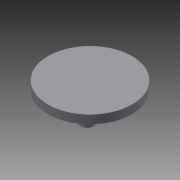
# Autodesk Inventor part: PSteg
Saved by Autodesk Inventor 2014 (Build 180170000, 170)
## iProperties
Created: 2013-05-23
Part Number: PSteg
Material: Generisch
Document SubType Name: Modeling
Designer: hartmann
Density: 1 g/cm^3
Appearance: Vorgabe
Author: hartmann
Autodesk Inventor part; units mm, degrees
ref_plane "YZ Plane" through (0, 0, 0) normal (1, 0, 0) x (0, 1, 0)
ref_plane "XZ Plane" through (0, 0, 0) normal (0, 1, 0) x (-1, 0, 0)
ref_plane "XY Plane" through (0, 0, 0) normal (0, 0, 1) x (1, 0, 0)
sketch "Skizze1" plane through (0, 0, 0) normal (0, 0, 1) x (1, 0, 0)
  arc A0 (1.0212, 1.5725) -> (1.1577, 2.2721) centre (-0.9647, 2.323) ccw projected
  arc A1 (1.1577, 2.2721) -> (0.9138, 2.3806) centre (0, 0) ccw projected
  arc A2 (0.9138, 2.3806) -> (0.4853, 1.8111) centre (2.3719, 0.8375) ccw projected
  arc A3 (0.4853, 1.8111) -> (0.2933, 1.8519) centre (0, 0) ccw projected
  arc A4 (0.2933, 1.8519) -> (0.1335, 2.5465) centre (-1.8262, 1.7298) ccw projected
  arc A5 (0.1335, 2.5465) -> (-0.1335, 2.5465) centre (0, 0) ccw projected
  arc A6 (-0.1335, 2.5465) -> (-0.2933, 1.8519) centre (1.8262, 1.7298) ccw projected
  arc A7 (-0.2933, 1.8519) -> (-0.4853, 1.8111) centre (0, 0) ccw projected
  arc A8 (-0.4853, 1.8111) -> (-0.9138, 2.3806) centre (-2.3719, 0.8375) ccw projected
  arc A9 (-0.9138, 2.3806) -> (-1.1577, 2.2721) centre (0, 0) ccw projected
  arc A10 (-1.1577, 2.2721) -> (-1.0212, 1.5725) centre (0.9647, 2.323) ccw projected
  arc A11 (-1.0212, 1.5725) -> (-1.18, 1.4571) centre (0, 0) ccw projected
  arc A12 (-1.18, 1.4571) -> (-1.8031, 1.8031) centre (-2.5074, -0.1996) ccw projected
  arc A13 (-1.8031, 1.8031) -> (-1.9817, 1.6048) centre (0, 0) ccw projected
  arc A14 (-1.9817, 1.6048) -> (-1.5725, 1.0212) centre (-0.0636, 2.5146) ccw projected
  arc A15 (-1.5725, 1.0212) -> (-1.6706, 0.8512) centre (0, 0) ccw projected
  arc A16 (-1.6706, 0.8512) -> (-2.3806, 0.9138) centre (-2.2095, -1.2022) ccw projected
  arc A17 (-2.3806, 0.9138) -> (-2.4631, 0.66) centre (0, 0) ccw projected
  arc A18 (-2.4631, 0.66) -> (-1.8519, 0.2933) centre (-1.0808, 2.2713) ccw projected
  arc A19 (-1.8519, 0.2933) -> (-1.8724, 0.0981) centre (0, 0) ccw projected
  arc A20 (-1.8724, 0.0981) -> (-2.5465, -0.1335) centre (-1.5295, -1.997) ccw projected
  arc A21 (-2.5465, -0.1335) -> (-2.5186, -0.3989) centre (0, 0) ccw projected
  arc A22 (-2.5186, -0.3989) -> (-1.8111, -0.4853) centre (-1.9112, 1.6353) ccw projected
  arc A23 (-1.8111, -0.4853) -> (-1.7505, -0.6719) centre (0, 0) ccw projected
  arc A24 (-1.7505, -0.6719) -> (-2.2721, -1.1577) centre (-0.585, -2.4464) ccw projected
  arc A25 (-2.2721, -1.1577) -> (-2.1386, -1.3888) centre (0, 0) ccw projected
  arc A26 (-2.1386, -1.3888) -> (-1.4571, -1.18) centre (-2.4111, 0.7166) ccw projected
  arc A27 (-1.4571, -1.18) -> (-1.3258, -1.3258) centre (0, 0) ccw projected
  arc A28 (-1.3258, -1.3258) -> (-1.6048, -1.9817) centre (0.4606, -2.4728) ccw projected
  arc A29 (-1.6048, -1.9817) -> (-1.3888, -2.1386) centre (0, 0) ccw projected
  arc A30 (-1.3888, -2.1386) -> (-0.8512, -1.6706) centre (-2.4942, -0.3261) ccw projected
  arc A31 (-0.8512, -1.6706) -> (-0.6719, -1.7505) centre (0, 0) ccw projected
  arc A32 (-0.6719, -1.7505) -> (-0.66, -2.4631) centre (1.4266, -2.0717) ccw projected
  arc A33 (-0.66, -2.4631) -> (-0.3989, -2.5186) centre (0, 0) ccw projected
  arc A34 (-0.3989, -2.5186) -> (-0.0981, -1.8724) centre (-2.1459, -1.3123) ccw projected
  arc A35 (-0.0981, -1.8724) -> (0.0981, -1.8724) centre (0, 0) ccw projected
  arc A36 (0.0981, -1.8724) -> (0.3989, -2.5186) centre (2.1459, -1.3123) ccw projected
  arc A37 (0.3989, -2.5186) -> (0.66, -2.4631) centre (0, 0) ccw projected
  arc A38 (0.66, -2.4631) -> (0.6719, -1.7505) centre (-1.4266, -2.0717) ccw projected
  arc A39 (0.6719, -1.7505) -> (0.8512, -1.6706) centre (0, 0) ccw projected
  arc A40 (0.8512, -1.6706) -> (1.3888, -2.1386) centre (2.4942, -0.3261) ccw projected
  arc A41 (1.3888, -2.1386) -> (1.6048, -1.9817) centre (0, 0) ccw projected
  arc A42 (1.6048, -1.9817) -> (1.3258, -1.3258) centre (-0.4606, -2.4728) ccw projected
  arc A43 (1.3258, -1.3258) -> (1.4571, -1.18) centre (0, 0) ccw projected
  arc A44 (1.4571, -1.18) -> (2.1386, -1.3888) centre (2.4111, 0.7166) ccw projected
  arc A45 (2.1386, -1.3888) -> (2.2721, -1.1577) centre (0, 0) ccw projected
  arc A46 (2.2721, -1.1577) -> (1.7505, -0.6719) centre (0.585, -2.4464) ccw projected
  arc A47 (1.7505, -0.6719) -> (1.8111, -0.4853) centre (0, 0) ccw projected
  arc A48 (1.8111, -0.4853) -> (2.5186, -0.3989) centre (1.9112, 1.6353) ccw projected
  arc A49 (2.5186, -0.3989) -> (2.5465, -0.1335) centre (0, 0) ccw projected
  arc A50 (2.5465, -0.1335) -> (1.8724, 0.0981) centre (1.5295, -1.997) ccw projected
  arc A51 (1.8724, 0.0981) -> (1.8519, 0.2933) centre (0, 0) ccw projected
  arc A52 (1.8519, 0.2933) -> (2.4631, 0.66) centre (1.0808, 2.2713) ccw projected
  arc A53 (2.4631, 0.66) -> (2.3806, 0.9138) centre (0, 0) ccw projected
  arc A54 (2.3806, 0.9138) -> (1.6706, 0.8512) centre (2.2095, -1.2022) ccw projected
  arc A55 (1.6706, 0.8512) -> (1.5725, 1.0212) centre (0, 0) ccw projected
  arc A56 (1.5725, 1.0212) -> (1.9817, 1.6048) centre (0.0636, 2.5146) ccw projected
  arc A57 (1.9817, 1.6048) -> (1.8031, 1.8031) centre (0, 0) ccw projected
  arc A58 (1.8031, 1.8031) -> (1.18, 1.4571) centre (2.5074, -0.1996) ccw projected
  arc A59 (1.18, 1.4571) -> (1.0212, 1.5725) centre (0, 0) ccw projected
  circle A60 centre (0, 0) radius 10
  dimension "d0" = 20
  constraints: 1 centre point, 1 coincident
  measures "d0" diameter of A60
extrude "Extrusion1" add sketch "Skizze1" along normal blind 2 contours A59 A58 A57 A56 A55 A54 A53 A52 A51 A50 A49 A48 A47 A46 A45 A44 A43 A42 A41 A40 A39 A38 A37 A36 A35 A34 A33 A32 A31 A30 A29 A28 A27 A26 A25 A24 A23 A22 A21 A20 A19 A18 A17 A16 A15 A14 A13 A12 A11 A10 A9 A8 A7 A6 A5 A4 A3 A2 A1 A0 | A60
sketch "Skizze2" plane through (0, 0, 0) normal (0, 0, -1) x (-1, 0, 0)
  circle A0 centre (-2.2201, 6.3744) radius 1.5 projected
  arc A1 (-5.5549, 8.8024) -> (-6.2431, 8.9928) centre (-6.6934, 6.0252) ccw projected
  arc A2 (-6.2431, 8.9928) -> (-6.3746, 8.7787) centre (-2.2201, 6.3744) ccw projected
  arc A3 (-6.3746, 8.7787) -> (-5.8936, 8.2509) centre (-3.9314, 10.5222) ccw projected
  arc A4 (-5.8936, 8.2509) -> (-5.9868, 8.056) centre (-2.2201, 6.3744) ccw projected
  arc A5 (-5.9868, 8.056) -> (-6.6996, 8.0992) centre (-6.5231, 5.1028) ccw projected
  arc A6 (-6.6996, 8.0992) -> (-6.7837, 7.8624) centre (-2.2201, 6.3744) ccw projected
  arc A7 (-6.7837, 7.8624) -> (-6.2035, 7.4461) centre (-4.7564, 10.0758) ccw projected
  arc A8 (-6.2035, 7.4461) -> (-6.2541, 7.2362) centre (-2.2201, 6.3744) ccw projected
  arc A9 (-6.2541, 7.2362) -> (-6.9603, 7.1301) centre (-6.1647, 4.236) ccw projected
  arc A10 (-6.9603, 7.1301) -> (-6.9933, 6.881) centre (-2.2201, 6.3744) ccw projected
  arc A11 (-6.9933, 6.881) -> (-6.3393, 6.5945) centre (-5.4705, 9.4676) ccw projected
  arc A12 (-6.3393, 6.5945) -> (-6.3451, 6.3786) centre (-2.2201, 6.3744) ccw projected
  arc A13 (-6.3451, 6.3786) -> (-7.0138, 6.1281) centre (-5.6339, 3.4626) ccw projected
  arc A14 (-7.0138, 6.1281) -> (-6.9944, 5.8775) centre (-2.2201, 6.3744) ccw projected
  arc A15 (-6.9944, 5.8775) -> (-6.295, 5.7333) centre (-6.0426, 8.7242) ccw projected
  arc A16 (-6.295, 5.7333) -> (-6.2559, 5.5209) centre (-2.2201, 6.3744) ccw projected
  arc A17 (-6.2559, 5.5209) -> (-6.8578, 5.1368) centre (-4.9539, 2.8165) ccw projected
  arc A18 (-6.8578, 5.1368) -> (-6.7867, 4.8958) centre (-2.2201, 6.3744) ccw projected
  arc A19 (-6.7867, 4.8958) -> (-6.0727, 4.9001) centre (-6.4476, 7.8781) ccw projected
  arc A20 (-6.0727, 4.9001) -> (-5.9902, 4.7005) centre (-2.2201, 6.3744) ccw projected
  arc A21 (-5.9902, 4.7005) -> (-6.4992, 4.1996) centre (-4.1544, 2.3259) ccw projected
  arc A22 (-6.4992, 4.1996) -> (-6.3795, 3.9787) centre (-2.2201, 6.3744) ccw projected
  arc A23 (-6.3795, 3.9787) -> (-5.6819, 4.1313) centre (-6.6678, 6.9663) ccw projected
  arc A24 (-5.6819, 4.1313) -> (-5.5598, 3.9532) centre (-2.2201, 6.3744) ccw projected
  arc A25 (-5.5598, 3.9532) -> (-5.9535, 3.3575) centre (-3.2704, 2.0122) ccw projected
  arc A26 (-5.9535, 3.3575) -> (-5.7905, 3.1662) centre (-2.2201, 6.3744) ccw projected
  arc A27 (-5.7905, 3.1662) -> (-5.1399, 3.4606) centre (-6.6937, 6.0286) ccw projected
  arc A28 (-5.1399, 3.4606) -> (-4.9834, 3.3118) centre (-2.2201, 6.3744) ccw projected
  arc A29 (-4.9834, 3.3118) -> (-5.2447, 2.6472) centre (-2.3404, 1.8891) ccw projected
  arc A30 (-5.2447, 2.6472) -> (-5.0455, 2.494) centre (-2.2201, 6.3744) ccw projected
  arc A31 (-5.0455, 2.494) -> (-4.4703, 2.9172) centre (-6.524, 5.1061) ccw projected
  arc A32 (-4.4703, 2.9172) -> (-4.2863, 2.8042) centre (-2.2201, 6.3744) ccw projected
  arc A33 (-4.2863, 2.8042) -> (-4.4036, 2.0998) centre (-1.4053, 1.9622) ccw projected
  arc A34 (-4.4036, 2.0998) -> (-4.1769, 1.9914) centre (-2.2201, 6.3744) ccw projected
  arc A35 (-4.1769, 1.9914) -> (-3.7023, 2.5249) centre (-6.1663, 4.239) ccw projected
  arc A36 (-3.7023, 2.5249) -> (-3.4988, 2.4526) centre (-2.2201, 6.3744) ccw projected
  arc A37 (-3.4988, 2.4526) -> (-3.4672, 1.7393) centre (-0.5057, 2.228) ccw projected
  arc A38 (-3.4672, 1.7393) -> (-3.2229, 1.6803) centre (-2.2201, 6.3744) ccw projected
  arc A39 (-3.2229, 1.6803) -> (-2.8696, 2.3009) centre (-5.6361, 3.4652) ccw projected
  arc A40 (-2.8696, 2.3009) -> (-2.6555, 2.2725) centre (-2.2201, 6.3744) ccw projected
  arc A41 (-2.6555, 2.2725) -> (-2.4762, 1.5813) centre (0.3189, 2.6751) ccw projected
  arc A42 (-2.4762, 1.5813) -> (-2.225, 1.5744) centre (-2.2201, 6.3744) ccw projected
  arc A43 (-2.225, 1.5744) -> (-2.0084, 2.2549) centre (-4.9566, 2.8186) ccw projected
  arc A44 (-2.0084, 2.2549) -> (-1.7931, 2.2716) centre (-2.2201, 6.3744) ccw projected
  arc A45 (-1.7931, 2.2716) -> (-1.4741, 1.6328) centre (1.0326, 3.2838) ccw projected
  arc A46 (-1.4741, 1.6328) -> (-1.2269, 1.6783) centre (-2.2201, 6.3744) ccw projected
  arc A47 (-1.2269, 1.6783) -> (-1.1566, 2.3889) centre (-4.1575, 2.3273) ccw projected
  arc A48 (-1.1566, 2.3889) -> (-0.9494, 2.45) centre (-2.2201, 6.3744) ccw projected
  arc A49 (-0.9494, 2.45) -> (-0.5045, 1.8915) centre (1.6041, 4.0276) ccw projected
  arc A50 (-0.5045, 1.8915) -> (-0.2723, 1.9874) centre (-2.2201, 6.3744) ccw projected
  arc A51 (-0.2723, 1.9874) -> (-0.3512, 2.6971) centre (-3.2737, 2.013) ccw projected
  arc A52 (-0.3512, 2.6971) -> (-0.1613, 2.8) centre (-2.2201, 6.3744) ccw projected
  arc A53 (-0.1613, 2.8) -> (0.39, 2.3462) centre (2.0084, 4.874) ccw projected
  arc A54 (0.39, 2.3462) -> (0.5973, 2.4883) centre (-2.2201, 6.3744) ccw projected
  arc A55 (0.5973, 2.4883) -> (0.3725, 3.1661) centre (-2.3439, 1.8892) ccw projected
  arc A56 (0.3725, 3.1661) -> (0.5369, 3.3062) centre (-2.2201, 6.3744) ccw projected
  arc A57 (0.5369, 3.3062) -> (1.1705, 2.9769) centre (2.228, 5.786) ccw projected
  arc A58 (1.1705, 2.9769) -> (1.3437, 3.159) centre (-2.2201, 6.3744) ccw projected
  arc A59 (1.3437, 3.159) -> (0.9829, 3.7752) centre (-1.4086, 1.9615) ccw projected
  arc A60 (0.9829, 3.7752) -> (1.1146, 3.9464) centre (-2.2201, 6.3744) ccw projected
  arc A61 (1.1146, 3.9464) -> (1.8028, 3.7561) centre (2.2531, 6.7236) ccw projected
  arc A62 (1.8028, 3.7561) -> (1.9343, 3.9702) centre (-2.2201, 6.3744) ccw projected
  arc A63 (1.9343, 3.9702) -> (1.4534, 4.498) centre (-0.5089, 2.2267) ccw projected
  arc A64 (1.4534, 4.498) -> (1.5465, 4.6928) centre (-2.2201, 6.3744) ccw projected
  arc A65 (1.5465, 4.6928) -> (2.2593, 4.6497) centre (2.0828, 7.6461) ccw projected
  arc A66 (2.2593, 4.6497) -> (2.3434, 4.8865) centre (-2.2201, 6.3744) ccw projected
  arc A67 (2.3434, 4.8865) -> (1.7632, 5.3028) centre (0.3161, 2.6731) ccw projected
  arc A68 (1.7632, 5.3028) -> (1.8138, 5.5127) centre (-2.2201, 6.3744) ccw projected
  arc A69 (1.8138, 5.5127) -> (2.52, 5.6187) centre (1.7244, 8.5129) ccw projected
  arc A70 (2.52, 5.6187) -> (2.553, 5.8679) centre (-2.2201, 6.3744) ccw projected
  arc A71 (2.553, 5.8679) -> (1.899, 6.1544) centre (1.0302, 3.2813) ccw projected
  arc A72 (1.899, 6.1544) -> (1.9049, 6.3703) centre (-2.2201, 6.3744) ccw projected
  arc A73 (1.9049, 6.3703) -> (2.5735, 6.6208) centre (1.1936, 9.2863) ccw projected
  arc A74 (2.5735, 6.6208) -> (2.5541, 6.8713) centre (-2.2201, 6.3744) ccw projected
  arc A75 (2.5541, 6.8713) -> (1.8547, 7.0156) centre (1.6023, 4.0247) ccw projected
  arc A76 (1.8547, 7.0156) -> (1.8156, 7.228) centre (-2.2201, 6.3744) ccw projected
  arc A77 (1.8156, 7.228) -> (2.4176, 7.6121) centre (0.5136, 9.9324) ccw projected
  arc A78 (2.4176, 7.6121) -> (2.3464, 7.8531) centre (-2.2201, 6.3744) ccw projected
  arc A79 (2.3464, 7.8531) -> (1.6324, 7.8488) centre (2.0073, 4.8708) ccw projected
  arc A80 (1.6324, 7.8488) -> (1.5499, 8.0484) centre (-2.2201, 6.3744) ccw projected
  arc A81 (1.5499, 8.0484) -> (2.0589, 8.5492) centre (-0.2859, 10.423) ccw projected
  arc A82 (2.0589, 8.5492) -> (1.9392, 8.7702) centre (-2.2201, 6.3744) ccw projected
  arc A83 (1.9392, 8.7702) -> (1.2416, 8.6176) centre (2.2275, 5.7826) ccw projected
  arc A84 (1.2416, 8.6176) -> (1.1195, 8.7957) centre (-2.2201, 6.3744) ccw projected
  arc A85 (1.1195, 8.7957) -> (1.5132, 9.3914) centre (-1.1699, 10.7367) ccw projected
  arc A86 (1.5132, 9.3914) -> (1.3502, 9.5826) centre (-2.2201, 6.3744) ccw projected
  arc A87 (1.3502, 9.5826) -> (0.6996, 9.2883) centre (2.2534, 6.7202) ccw projected
  arc A88 (0.6996, 9.2883) -> (0.5431, 9.4371) centre (-2.2201, 6.3744) ccw projected
  arc A89 (0.5431, 9.4371) -> (0.8044, 10.1017) centre (-2.0998, 10.8597) ccw projected
  arc A90 (0.8044, 10.1017) -> (0.6052, 10.2549) centre (-2.2201, 6.3744) ccw projected
  arc A91 (0.6052, 10.2549) -> (0.03, 9.8317) centre (2.0838, 7.6428) ccw projected
  arc A92 (0.03, 9.8317) -> (-0.154, 9.9447) centre (-2.2201, 6.3744) ccw projected
  arc A93 (-0.154, 9.9447) -> (-0.0367, 10.6491) centre (-3.035, 10.7867) ccw projected
  arc A94 (-0.0367, 10.6491) -> (-0.2634, 10.7575) centre (-2.2201, 6.3744) ccw projected
  arc A95 (-0.2634, 10.7575) -> (-0.738, 10.224) centre (1.726, 8.5099) ccw projected
  arc A96 (-0.738, 10.224) -> (-0.9415, 10.2962) centre (-2.2201, 6.3744) ccw projected
  arc A97 (-0.9415, 10.2962) -> (-0.9731, 11.0096) centre (-3.9346, 10.5209) ccw projected
  arc A98 (-0.9731, 11.0096) -> (-1.2174, 11.0685) centre (-2.2201, 6.3744) ccw projected
  arc A99 (-1.2174, 11.0685) -> (-1.5707, 10.448) centre (1.1958, 9.2837) ccw projected
  arc A100 (-1.5707, 10.448) -> (-1.7848, 10.4764) centre (-2.2201, 6.3744) ccw projected
  arc A101 (-1.7848, 10.4764) -> (-1.9641, 11.1676) centre (-4.7592, 10.0738) ccw projected
  arc A102 (-1.9641, 11.1676) -> (-2.2153, 11.1744) centre (-2.2201, 6.3744) ccw projected
  arc A103 (-2.2153, 11.1744) -> (-2.4319, 10.494) centre (0.5163, 9.9303) ccw projected
  arc A104 (-2.4319, 10.494) -> (-2.6472, 10.4773) centre (-2.2201, 6.3744) ccw projected
  arc A105 (-2.6472, 10.4773) -> (-2.9662, 11.1161) centre (-5.4729, 9.4651) ccw projected
  arc A106 (-2.9662, 11.1161) -> (-3.2134, 11.0706) centre (-2.2201, 6.3744) ccw projected
  arc A107 (-3.2134, 11.0706) -> (-3.2837, 10.36) centre (-0.2828, 10.4216) ccw projected
  arc A108 (-3.2837, 10.36) -> (-3.4909, 10.2988) centre (-2.2201, 6.3744) ccw projected
  arc A109 (-3.4909, 10.2988) -> (-3.9358, 10.8574) centre (-6.0444, 8.7213) ccw projected
  arc A110 (-3.9358, 10.8574) -> (-4.168, 10.7614) centre (-2.2201, 6.3744) ccw projected
  arc A111 (-4.168, 10.7614) -> (-4.0891, 10.0517) centre (-1.1666, 10.7359) ccw projected
  arc A112 (-4.0891, 10.0517) -> (-4.279, 9.9489) centre (-2.2201, 6.3744) ccw projected
  arc A113 (-4.279, 9.9489) -> (-4.8303, 10.4027) centre (-6.4487, 7.8749) ccw projected
  arc A114 (-4.8303, 10.4027) -> (-5.0376, 10.2606) centre (-2.2201, 6.3744) ccw projected
  arc A115 (-5.0376, 10.2606) -> (-4.8128, 9.5828) centre (-2.0964, 10.8596) ccw projected
  arc A116 (-4.8128, 9.5828) -> (-4.9772, 9.4427) centre (-2.2201, 6.3744) ccw projected
  arc A117 (-4.9772, 9.4427) -> (-5.6108, 9.772) centre (-6.6683, 6.9629) ccw projected
  arc A118 (-5.6108, 9.772) -> (-5.784, 9.5899) centre (-2.2201, 6.3744) ccw projected
  arc A119 (-5.784, 9.5899) -> (-5.4232, 8.9736) centre (-3.0317, 10.7873) ccw projected
  arc A120 (-5.4232, 8.9736) -> (-5.5549, 8.8024) centre (-2.2201, 6.3744) ccw projected
  circle A121 centre (-4.4104, -5.1099) radius 1.5 projected
  arc A122 (-4.8457, -9.2119) -> (-4.6664, -9.9031) centre (-1.8713, -8.8093) ccw projected
  arc A123 (-4.6664, -9.9031) -> (-4.4152, -9.9099) centre (-4.4104, -5.1099) ccw projected
  arc A124 (-4.4152, -9.9099) -> (-4.1986, -9.2295) centre (-7.1468, -8.6658) ccw projected
  arc A125 (-4.1986, -9.2295) -> (-3.9833, -9.2128) centre (-4.4104, -5.1099) ccw projected
  arc A126 (-3.9833, -9.2128) -> (-3.6643, -9.8516) centre (-1.1576, -8.2006) ccw projected
  arc A127 (-3.6643, -9.8516) -> (-3.4171, -9.806) centre (-4.4104, -5.1099) ccw projected
  arc A128 (-3.4171, -9.806) -> (-3.3468, -9.0954) centre (-6.3477, -9.157) ccw projected
  arc A129 (-3.3468, -9.0954) -> (-3.1396, -9.0343) centre (-4.4104, -5.1099) ccw projected
  arc A130 (-3.1396, -9.0343) -> (-2.6947, -9.5929) centre (-0.5861, -7.4568) ccw projected
  arc A131 (-2.6947, -9.5929) -> (-2.4625, -9.4969) centre (-4.4104, -5.1099) ccw projected
  arc A132 (-2.4625, -9.4969) -> (-2.5414, -8.7872) centre (-5.4639, -9.4714) ccw projected
  arc A133 (-2.5414, -8.7872) -> (-2.3515, -8.6844) centre (-4.4104, -5.1099) ccw projected
  arc A134 (-2.3515, -8.6844) -> (-1.8002, -9.1382) centre (-0.1818, -6.6104) ccw projected
  arc A135 (-1.8002, -9.1382) -> (-1.5929, -8.9961) centre (-4.4104, -5.1099) ccw projected
  arc A136 (-1.5929, -8.9961) -> (-1.8177, -8.3183) centre (-4.5341, -9.5951) ccw projected
  arc A137 (-1.8177, -8.3183) -> (-1.6533, -8.1782) centre (-4.4104, -5.1099) ccw projected
  arc A138 (-1.6533, -8.1782) -> (-1.0197, -8.5075) centre (0.0378, -5.6984) ccw projected
  arc A139 (-1.0197, -8.5075) -> (-0.8465, -8.3254) centre (-4.4104, -5.1099) ccw projected
  arc A140 (-0.8465, -8.3254) -> (-1.2073, -7.7091) centre (-3.5988, -9.5228) ccw projected
  arc A141 (-1.2073, -7.7091) -> (-1.0756, -7.5379) centre (-4.4104, -5.1099) ccw projected
  arc A142 (-1.0756, -7.5379) -> (-0.3874, -7.7283) centre (0.0629, -4.7607) ccw projected
  arc A143 (-0.3874, -7.7283) -> (-0.2559, -7.5141) centre (-4.4104, -5.1099) ccw projected
  arc A144 (-0.2559, -7.5141) -> (-0.7369, -6.9864) centre (-2.6991, -9.2577) ccw projected
  arc A145 (-0.7369, -6.9864) -> (-0.6437, -6.7915) centre (-4.4104, -5.1099) ccw projected
  arc A146 (-0.6437, -6.7915) -> (0.0691, -6.8346) centre (-0.1074, -3.8383) ccw projected
  arc A147 (0.0691, -6.8346) -> (0.1532, -6.5978) centre (-4.4104, -5.1099) ccw projected
  arc A148 (0.1532, -6.5978) -> (-0.427, -6.1816) centre (-1.8741, -8.8112) ccw projected
  arc A149 (-0.427, -6.1816) -> (-0.3764, -5.9717) centre (-4.4104, -5.1099) ccw projected
  arc A150 (-0.3764, -5.9717) -> (0.3298, -5.8656) centre (-0.4658, -2.9715) ccw projected
  arc A151 (0.3298, -5.8656) -> (0.3628, -5.6165) centre (-4.4104, -5.1099) ccw projected
  arc A152 (0.3628, -5.6165) -> (-0.2912, -5.33) centre (-1.16, -8.203) ccw projected
  arc A153 (-0.2912, -5.33) -> (-0.2854, -5.1141) centre (-4.4104, -5.1099) ccw projected
  arc A154 (-0.2854, -5.1141) -> (0.3833, -4.8636) centre (-0.9966, -2.1981) ccw projected
  arc A155 (0.3833, -4.8636) -> (0.3639, -4.613) centre (-4.4104, -5.1099) ccw projected
  arc A156 (0.3639, -4.613) -> (-0.3355, -4.4688) centre (-0.5879, -7.4597) ccw projected
  arc A157 (-0.3355, -4.4688) -> (-0.3746, -4.2564) centre (-4.4104, -5.1099) ccw projected
  arc A158 (-0.3746, -4.2564) -> (0.2274, -3.8723) centre (-1.6766, -1.552) ccw projected
  arc A159 (0.2274, -3.8723) -> (0.1562, -3.6313) centre (-4.4104, -5.1099) ccw projected
  arc A160 (0.1562, -3.6313) -> (-0.5578, -3.6356) centre (-0.1829, -6.6136) ccw projected
  arc A161 (-0.5578, -3.6356) -> (-0.6403, -3.436) centre (-4.4104, -5.1099) ccw projected
  arc A162 (-0.6403, -3.436) -> (-0.1313, -2.9351) centre (-2.4761, -1.0613) ccw projected
  arc A163 (-0.1313, -2.9351) -> (-0.251, -2.7141) centre (-4.4104, -5.1099) ccw projected
  arc A164 (-0.251, -2.7141) -> (-0.9486, -2.8668) centre (0.0373, -5.7018) ccw projected
  arc A165 (-0.9486, -2.8668) -> (-1.0707, -2.6887) centre (-4.4104, -5.1099) ccw projected
  arc A166 (-1.0707, -2.6887) -> (-0.677, -2.093) centre (-3.3601, -0.7477) ccw projected
  arc A167 (-0.677, -2.093) -> (-0.84, -1.9017) centre (-4.4104, -5.1099) ccw projected
  arc A168 (-0.84, -1.9017) -> (-1.4906, -2.1961) centre (0.0632, -4.7641) ccw projected
  arc A169 (-1.4906, -2.1961) -> (-1.6471, -2.0473) centre (-4.4104, -5.1099) ccw projected
  arc A170 (-1.6471, -2.0473) -> (-1.3858, -1.3827) centre (-4.29, -0.6246) ccw projected
  arc A171 (-1.3858, -1.3827) -> (-1.585, -1.2295) centre (-4.4104, -5.1099) ccw projected
  arc A172 (-1.585, -1.2295) -> (-2.1602, -1.6527) centre (-0.1064, -3.8416) ccw projected
  arc A173 (-2.1602, -1.6527) -> (-2.3442, -1.5397) centre (-4.4104, -5.1099) ccw projected
  arc A174 (-2.3442, -1.5397) -> (-2.2269, -0.8353) centre (-5.2252, -0.6976) ccw projected
  arc A175 (-2.2269, -0.8353) -> (-2.4536, -0.7269) centre (-4.4104, -5.1099) ccw projected
  arc A176 (-2.4536, -0.7269) -> (-2.9282, -1.2604) centre (-0.4642, -2.9745) ccw projected
  arc A177 (-2.9282, -1.2604) -> (-3.1317, -1.1881) centre (-4.4104, -5.1099) ccw projected
  arc A178 (-3.1317, -1.1881) -> (-3.1633, -0.4747) centre (-6.1248, -0.9635) ccw projected
  arc A179 (-3.1633, -0.4747) -> (-3.4076, -0.4158) centre (-4.4104, -5.1099) ccw projected
  arc A180 (-3.4076, -0.4158) -> (-3.7609, -1.0364) centre (-0.9944, -2.2007) ccw projected
  arc A181 (-3.7609, -1.0364) -> (-3.975, -1.008) centre (-4.4104, -5.1099) ccw projected
  arc A182 (-3.975, -1.008) -> (-4.1543, -0.3168) centre (-6.9494, -1.4105) ccw projected
  arc A183 (-4.1543, -0.3168) -> (-4.4055, -0.3099) centre (-4.4104, -5.1099) ccw projected
  arc A184 (-4.4055, -0.3099) -> (-4.6221, -0.9904) centre (-1.6739, -1.554) ccw projected
  arc A185 (-4.6221, -0.9904) -> (-4.8374, -1.0071) centre (-4.4104, -5.1099) ccw projected
  arc A186 (-4.8374, -1.0071) -> (-5.1564, -0.3683) centre (-7.6631, -2.0193) ccw projected
  arc A187 (-5.1564, -0.3683) -> (-5.4036, -0.4138) centre (-4.4104, -5.1099) ccw projected
  arc A188 (-5.4036, -0.4138) -> (-5.4739, -1.1244) centre (-2.473, -1.0628) ccw projected
  arc A189 (-5.4739, -1.1244) -> (-5.6811, -1.1855) centre (-4.4104, -5.1099) ccw projected
  arc A190 (-5.6811, -1.1855) -> (-6.126, -0.627) centre (-8.2346, -2.7631) ccw projected
  arc A191 (-6.126, -0.627) -> (-6.3582, -0.7229) centre (-4.4104, -5.1099) ccw projected
  arc A192 (-6.3582, -0.7229) -> (-6.2793, -1.4326) centre (-3.3568, -0.7485) ccw projected
  arc A193 (-6.2793, -1.4326) -> (-6.4692, -1.5355) centre (-4.4104, -5.1099) ccw projected
  arc A194 (-6.4692, -1.5355) -> (-7.0205, -1.0817) centre (-8.6389, -3.6095) ccw projected
  arc A195 (-7.0205, -1.0817) -> (-7.2278, -1.2238) centre (-4.4104, -5.1099) ccw projected
  arc A196 (-7.2278, -1.2238) -> (-7.003, -1.9016) centre (-4.2866, -0.6247) ccw projected
  arc A197 (-7.003, -1.9016) -> (-7.1674, -2.0417) centre (-4.4104, -5.1099) ccw projected
  arc A198 (-7.1674, -2.0417) -> (-7.801, -1.7124) centre (-8.8585, -4.5214) ccw projected
  arc A199 (-7.801, -1.7124) -> (-7.9742, -1.8945) centre (-4.4104, -5.1099) ccw projected
  arc A200 (-7.9742, -1.8945) -> (-7.6134, -2.5107) centre (-5.2219, -0.697) ccw projected
  arc A201 (-7.6134, -2.5107) -> (-7.7451, -2.6819) centre (-4.4104, -5.1099) ccw projected
  arc A202 (-7.7451, -2.6819) -> (-8.4333, -2.4916) centre (-8.8836, -5.4591) ccw projected
  arc A203 (-8.4333, -2.4916) -> (-8.5648, -2.7057) centre (-4.4104, -5.1099) ccw projected
  arc A204 (-8.5648, -2.7057) -> (-8.0839, -3.2335) centre (-6.1216, -0.9622) ccw projected
  arc A205 (-8.0839, -3.2335) -> (-8.177, -3.4283) centre (-4.4104, -5.1099) ccw projected
  arc A206 (-8.177, -3.4283) -> (-8.8898, -3.3852) centre (-8.7133, -6.3815) ccw projected
  arc A207 (-8.8898, -3.3852) -> (-8.9739, -3.622) centre (-4.4104, -5.1099) ccw projected
  arc A208 (-8.9739, -3.622) -> (-8.3937, -4.0383) centre (-6.9466, -1.4086) ccw projected
  arc A209 (-8.3937, -4.0383) -> (-8.4443, -4.2482) centre (-4.4104, -5.1099) ccw projected
  arc A210 (-8.4443, -4.2482) -> (-9.1505, -4.3542) centre (-8.3549, -7.2484) ccw projected
  arc A211 (-9.1505, -4.3542) -> (-9.1835, -4.6033) centre (-4.4104, -5.1099) ccw projected
  arc A212 (-9.1835, -4.6033) -> (-8.5295, -4.8899) centre (-7.6607, -2.0168) ccw projected
  arc A213 (-8.5295, -4.8899) -> (-8.5353, -5.1057) centre (-4.4104, -5.1099) ccw projected
  arc A214 (-8.5353, -5.1057) -> (-9.204, -5.3563) centre (-7.8241, -8.0218) ccw projected
  arc A215 (-9.204, -5.3563) -> (-9.1846, -5.6068) centre (-4.4104, -5.1099) ccw projected
  arc A216 (-9.1846, -5.6068) -> (-8.4852, -5.7511) centre (-8.2328, -2.7602) ccw projected
  arc A217 (-8.4852, -5.7511) -> (-8.4461, -5.9635) centre (-4.4104, -5.1099) ccw projected
  arc A218 (-8.4461, -5.9635) -> (-9.0481, -6.3475) centre (-7.1441, -8.6679) ccw projected
  arc A219 (-9.0481, -6.3475) -> (-8.9769, -6.5886) centre (-4.4104, -5.1099) ccw projected
  arc A220 (-8.9769, -6.5886) -> (-8.2629, -6.5843) centre (-8.6378, -3.6063) ccw projected
  arc A221 (-8.2629, -6.5843) -> (-8.1804, -6.7839) centre (-4.4104, -5.1099) ccw projected
  arc A222 (-8.1804, -6.7839) -> (-8.6894, -7.2847) centre (-6.3446, -9.1585) ccw projected
  arc A223 (-8.6894, -7.2847) -> (-8.5697, -7.5057) centre (-4.4104, -5.1099) ccw projected
  arc A224 (-8.5697, -7.5057) -> (-7.8721, -7.353) centre (-8.858, -4.5181) ccw projected
  arc A225 (-7.8721, -7.353) -> (-7.75, -7.5311) centre (-4.4104, -5.1099) ccw projected
  arc A226 (-7.75, -7.5311) -> (-8.1437, -8.1269) centre (-5.4606, -9.4722) ccw projected
  arc A227 (-8.1437, -8.1269) -> (-7.9807, -8.3181) centre (-4.4104, -5.1099) ccw projected
  arc A228 (-7.9807, -8.3181) -> (-7.3301, -8.0238) centre (-8.8839, -5.4557) ccw projected
  arc A229 (-7.3301, -8.0238) -> (-7.1736, -8.1726) centre (-4.4104, -5.1099) ccw projected
  arc A230 (-7.1736, -8.1726) -> (-7.4349, -8.8372) centre (-4.5307, -9.5952) ccw projected
  arc A231 (-7.4349, -8.8372) -> (-7.2357, -8.9903) centre (-4.4104, -5.1099) ccw projected
  arc A232 (-7.2357, -8.9903) -> (-6.6605, -8.5672) centre (-8.7143, -6.3783) ccw projected
  arc A233 (-6.6605, -8.5672) -> (-6.4765, -8.6802) centre (-4.4104, -5.1099) ccw projected
  arc A234 (-6.4765, -8.6802) -> (-6.5938, -9.3845) centre (-3.5955, -9.5222) ccw projected
  arc A235 (-6.5938, -9.3845) -> (-6.3671, -9.493) centre (-4.4104, -5.1099) ccw projected
  arc A236 (-6.3671, -9.493) -> (-5.8925, -8.9594) centre (-8.3565, -7.2454) ccw projected
  arc A237 (-5.8925, -8.9594) -> (-5.689, -9.0317) centre (-4.4104, -5.1099) ccw projected
  arc A238 (-5.689, -9.0317) -> (-5.6574, -9.7451) centre (-2.6959, -9.2564) ccw projected
  arc A239 (-5.6574, -9.7451) -> (-5.4131, -9.804) centre (-4.4104, -5.1099) ccw projected
  arc A240 (-5.4131, -9.804) -> (-5.0598, -9.1835) centre (-7.8263, -8.0192) ccw projected
  arc A241 (-5.0598, -9.1835) -> (-4.8457, -9.2119) centre (-4.4104, -5.1099) ccw projected
  circle A242 centre (6.6305, -1.2645) radius 1.5 projected
  arc A243 (10.4006, 0.4094) -> (10.9095, 0.9103) centre (8.5647, 2.7841) ccw projected
  arc A244 (10.9095, 0.9103) -> (10.7899, 1.1313) centre (6.6305, -1.2645) ccw projected
  arc A245 (10.7899, 1.1313) -> (10.0923, 0.9786) centre (11.0782, -1.8564) ccw projected
  arc A246 (10.0923, 0.9786) -> (9.9702, 1.1567) centre (6.6305, -1.2645) ccw projected
  arc A247 (9.9702, 1.1567) -> (10.3639, 1.7524) centre (7.6807, 3.0977) ccw projected
  arc A248 (10.3639, 1.7524) -> (10.2009, 1.9437) centre (6.6305, -1.2645) ccw projected
  arc A249 (10.2009, 1.9437) -> (9.5503, 1.6493) centre (11.1041, -0.9187) ccw projected
  arc A250 (9.5503, 1.6493) -> (9.3938, 1.7982) centre (6.6305, -1.2645) ccw projected
  arc A251 (9.3938, 1.7982) -> (9.655, 2.4627) centre (6.7508, 3.2208) ccw projected
  arc A252 (9.655, 2.4627) -> (9.4558, 2.6159) centre (6.6305, -1.2645) ccw projected
  arc A253 (9.4558, 2.6159) -> (8.8806, 2.1927) centre (10.9344, 0.0038) ccw projected
  arc A254 (8.8806, 2.1927) -> (8.6966, 2.3057) centre (6.6305, -1.2645) ccw projected
  arc A255 (8.6966, 2.3057) -> (8.814, 3.0101) centre (5.8156, 3.1478) ccw projected
  arc A256 (8.814, 3.0101) -> (8.5873, 3.1185) centre (6.6305, -1.2645) ccw projected
  arc A257 (8.5873, 3.1185) -> (8.1127, 2.585) centre (10.5766, 0.8709) ccw projected
  arc A258 (8.1127, 2.585) -> (7.9092, 2.6573) centre (6.6305, -1.2645) ccw projected
  arc A259 (7.9092, 2.6573) -> (7.8775, 3.3707) centre (4.9161, 2.8819) ccw projected
  arc A260 (7.8775, 3.3707) -> (7.6332, 3.4296) centre (6.6305, -1.2645) ccw projected
  arc A261 (7.6332, 3.4296) -> (7.2799, 2.809) centre (10.0464, 1.6447) ccw projected
  arc A262 (7.2799, 2.809) -> (7.0658, 2.8374) centre (6.6305, -1.2645) ccw projected
  arc A263 (7.0658, 2.8374) -> (6.8866, 3.5286) centre (4.0914, 2.4349) ccw projected
  arc A264 (6.8866, 3.5286) -> (6.6354, 3.5355) centre (6.6305, -1.2645) ccw projected
  arc A265 (6.6354, 3.5355) -> (6.4188, 2.855) centre (9.3669, 2.2914) ccw projected
  arc A266 (6.4188, 2.855) -> (6.2035, 2.8383) centre (6.6305, -1.2645) ccw projected
  arc A267 (6.2035, 2.8383) -> (5.8844, 3.4771) centre (3.3778, 1.8261) ccw projected
  arc A268 (5.8844, 3.4771) -> (5.6373, 3.4316) centre (6.6305, -1.2645) ccw projected
  arc A269 (5.6373, 3.4316) -> (5.5669, 2.721) centre (8.5678, 2.7826) ccw projected
  arc A270 (5.5669, 2.721) -> (5.3598, 2.6599) centre (6.6305, -1.2645) ccw projected
  arc A271 (5.3598, 2.6599) -> (4.9149, 3.2184) centre (2.8063, 1.0823) ccw projected
  arc A272 (4.9149, 3.2184) -> (4.6826, 3.1225) centre (6.6305, -1.2645) ccw projected
  arc A273 (4.6826, 3.1225) -> (4.7615, 2.4128) centre (7.684, 3.0969) ccw projected
  arc A274 (4.7615, 2.4128) -> (4.5716, 2.3099) centre (6.6305, -1.2645) ccw projected
  arc A275 (4.5716, 2.3099) -> (4.0203, 2.7638) centre (2.4019, 0.2359) ccw projected
  arc A276 (4.0203, 2.7638) -> (3.8131, 2.6216) centre (6.6305, -1.2645) ccw projected
  arc A277 (3.8131, 2.6216) -> (4.0378, 1.9438) centre (6.7542, 3.2207) ccw projected
  arc A278 (4.0378, 1.9438) -> (3.8734, 1.8038) centre (6.6305, -1.2645) ccw projected
  arc A279 (3.8734, 1.8038) -> (3.2398, 2.133) centre (2.1824, -0.676) ccw projected
  arc A280 (3.2398, 2.133) -> (3.0667, 1.9509) centre (6.6305, -1.2645) ccw projected
  arc A281 (3.0667, 1.9509) -> (3.4274, 1.3347) centre (5.819, 3.1484) ccw projected
  arc A282 (3.4274, 1.3347) -> (3.2958, 1.1635) centre (6.6305, -1.2645) ccw projected
  arc A283 (3.2958, 1.1635) -> (2.6075, 1.3538) centre (2.1572, -1.6137) ccw projected
  arc A284 (2.6075, 1.3538) -> (2.476, 1.1397) centre (6.6305, -1.2645) ccw projected
  arc A285 (2.476, 1.1397) -> (2.957, 0.6119) centre (4.9192, 2.8832) ccw projected
  arc A286 (2.957, 0.6119) -> (2.8638, 0.4171) centre (6.6305, -1.2645) ccw projected
  arc A287 (2.8638, 0.4171) -> (2.1511, 0.4602) centre (2.3276, -2.5361) ccw projected
  arc A288 (2.1511, 0.4602) -> (2.0669, 0.2234) centre (6.6305, -1.2645) ccw projected
  arc A289 (2.0669, 0.2234) -> (2.6471, -0.1928) centre (4.0942, 2.4368) ccw projected
  arc A290 (2.6471, -0.1928) -> (2.5965, -0.4028) centre (6.6305, -1.2645) ccw projected
  arc A291 (2.5965, -0.4028) -> (1.8904, -0.5088) centre (2.686, -3.403) ccw projected
  arc A292 (1.8904, -0.5088) -> (1.8573, -0.7579) centre (6.6305, -1.2645) ccw projected
  arc A293 (1.8573, -0.7579) -> (2.5114, -1.0444) centre (3.3801, 1.8286) ccw projected
  arc A294 (2.5114, -1.0444) -> (2.5055, -1.2603) centre (6.6305, -1.2645) ccw projected
  arc A295 (2.5055, -1.2603) -> (1.8368, -1.5109) centre (3.2168, -4.1764) ccw projected
  arc A296 (1.8368, -1.5109) -> (1.8563, -1.7614) centre (6.6305, -1.2645) ccw projected
  arc A297 (1.8563, -1.7614) -> (2.5556, -1.9057) centre (2.8081, 1.0852) ccw projected
  arc A298 (2.5556, -1.9057) -> (2.5948, -2.1181) centre (6.6305, -1.2645) ccw projected
  arc A299 (2.5948, -2.1181) -> (1.9928, -2.5021) centre (3.8968, -4.8225) ccw projected
  arc A300 (1.9928, -2.5021) -> (2.0639, -2.7432) centre (6.6305, -1.2645) ccw projected
  arc A301 (2.0639, -2.7432) -> (2.778, -2.7389) centre (2.4031, 0.2391) ccw projected
  arc A302 (2.778, -2.7389) -> (2.8604, -2.9385) centre (6.6305, -1.2645) ccw projected
  arc A303 (2.8604, -2.9385) -> (2.3515, -3.4393) centre (4.6963, -5.3131) ccw projected
  arc A304 (2.3515, -3.4393) -> (2.4711, -3.6603) centre (6.6305, -1.2645) ccw projected
  arc A305 (2.4711, -3.6603) -> (3.1687, -3.5076) centre (2.1828, -0.6727) ccw projected
  arc A306 (3.1687, -3.5076) -> (3.2908, -3.6857) centre (6.6305, -1.2645) ccw projected
  arc A307 (3.2908, -3.6857) -> (2.8971, -4.2815) centre (5.5803, -5.6268) ccw projected
  arc A308 (2.8971, -4.2815) -> (3.0601, -4.4727) centre (6.6305, -1.2645) ccw projected
  arc A309 (3.0601, -4.4727) -> (3.7107, -4.1784) centre (2.1569, -1.6103) ccw projected
  arc A310 (3.7107, -4.1784) -> (3.8672, -4.3272) centre (6.6305, -1.2645) ccw projected
  arc A311 (3.8672, -4.3272) -> (3.606, -4.9917) centre (6.5102, -5.7498) ccw projected
  arc A312 (3.606, -4.9917) -> (3.8052, -5.1449) centre (6.6305, -1.2645) ccw projected
  arc A313 (3.8052, -5.1449) -> (4.3804, -4.7217) centre (2.3266, -2.5329) ccw projected
  arc A314 (4.3804, -4.7217) -> (4.5644, -4.8348) centre (6.6305, -1.2645) ccw projected
  arc A315 (4.5644, -4.8348) -> (4.447, -5.5391) centre (7.4454, -5.6768) ccw projected
  arc A316 (4.447, -5.5391) -> (4.6737, -5.6475) centre (6.6305, -1.2645) ccw projected
  arc A317 (4.6737, -5.6475) -> (5.1483, -5.114) centre (2.6843, -3.4) ccw projected
  arc A318 (5.1483, -5.114) -> (5.3518, -5.1863) centre (6.6305, -1.2645) ccw projected
  arc A319 (5.3518, -5.1863) -> (5.3835, -5.8997) centre (8.3449, -5.411) ccw projected
  arc A320 (5.3835, -5.8997) -> (5.6278, -5.9586) centre (6.6305, -1.2645) ccw projected
  arc A321 (5.6278, -5.9586) -> (5.9811, -5.3381) centre (3.2146, -4.1738) ccw projected
  arc A322 (5.9811, -5.3381) -> (6.1952, -5.3665) centre (6.6305, -1.2645) ccw projected
  arc A323 (6.1952, -5.3665) -> (6.3744, -6.0577) centre (9.1696, -4.9639) ccw projected
  arc A324 (6.3744, -6.0577) -> (6.6256, -6.0645) centre (6.6305, -1.2645) ccw projected
  arc A325 (6.6256, -6.0645) -> (6.8422, -5.3841) centre (3.8941, -4.8204) ccw projected
  arc A326 (6.8422, -5.3841) -> (7.0575, -5.3674) centre (6.6305, -1.2645) ccw projected
  arc A327 (7.0575, -5.3674) -> (7.3766, -6.0062) centre (9.8832, -4.3552) ccw projected
  arc A328 (7.3766, -6.0062) -> (7.6237, -5.9606) centre (6.6305, -1.2645) ccw projected
  arc A329 (7.6237, -5.9606) -> (7.6941, -5.25) centre (4.6932, -5.3116) ccw projected
  arc A330 (7.6941, -5.25) -> (7.9012, -5.1889) centre (6.6305, -1.2645) ccw projected
  arc A331 (7.9012, -5.1889) -> (8.3461, -5.7474) centre (10.4547, -3.6113) ccw projected
  arc A332 (8.3461, -5.7474) -> (8.5784, -5.6515) centre (6.6305, -1.2645) ccw projected
  arc A333 (8.5784, -5.6515) -> (8.4995, -4.9418) centre (5.577, -5.626) ccw projected
  arc A334 (8.4995, -4.9418) -> (8.6894, -4.839) centre (6.6305, -1.2645) ccw projected
  arc A335 (8.6894, -4.839) -> (9.2407, -5.2928) centre (10.8591, -2.765) ccw projected
  arc A336 (9.2407, -5.2928) -> (9.4479, -5.1507) centre (6.6305, -1.2645) ccw projected
  arc A337 (9.4479, -5.1507) -> (9.2232, -4.4729) centre (6.5068, -5.7497) ccw projected
  arc A338 (9.2232, -4.4729) -> (9.3875, -4.3328) centre (6.6305, -1.2645) ccw projected
  arc A339 (9.3875, -4.3328) -> (10.0212, -4.6621) centre (11.0786, -1.853) ccw projected
  arc A340 (10.0212, -4.6621) -> (10.1943, -4.48) centre (6.6305, -1.2645) ccw projected
  arc A341 (10.1943, -4.48) -> (9.8336, -3.8637) centre (7.442, -5.6774) ccw projected
  arc A342 (9.8336, -3.8637) -> (9.9652, -3.6925) centre (6.6305, -1.2645) ccw projected
  arc A343 (9.9652, -3.6925) -> (10.6535, -3.8829) centre (11.1038, -0.9153) ccw projected
  arc A344 (10.6535, -3.8829) -> (10.785, -3.6687) centre (6.6305, -1.2645) ccw projected
  arc A345 (10.785, -3.6687) -> (10.304, -3.141) centre (8.3418, -5.4123) ccw projected
  arc A346 (10.304, -3.141) -> (10.3972, -2.9461) centre (6.6305, -1.2645) ccw projected
  arc A347 (10.3972, -2.9461) -> (11.1099, -2.9892) centre (10.9334, 0.0071) ccw projected
  arc A348 (11.1099, -2.9892) -> (11.1941, -2.7524) centre (6.6305, -1.2645) ccw projected
  arc A349 (11.1941, -2.7524) -> (10.6139, -2.3362) centre (9.1667, -4.9658) ccw projected
  arc A350 (10.6139, -2.3362) -> (10.6645, -2.1262) centre (6.6305, -1.2645) ccw projected
  arc A351 (10.6645, -2.1262) -> (11.3706, -2.0202) centre (10.575, 0.8739) ccw projected
  arc A352 (11.3706, -2.0202) -> (11.4037, -1.7711) centre (6.6305, -1.2645) ccw projected
  arc A353 (11.4037, -1.7711) -> (10.7496, -1.4846) centre (9.8809, -4.3576) ccw projected
  arc A354 (10.7496, -1.4846) -> (10.7555, -1.2687) centre (6.6305, -1.2645) ccw projected
  arc A355 (10.7555, -1.2687) -> (11.4242, -1.0182) centre (10.0442, 1.6473) ccw projected
  arc A356 (11.4242, -1.0182) -> (11.4047, -0.7676) centre (6.6305, -1.2645) ccw projected
  arc A357 (11.4047, -0.7676) -> (10.7054, -0.6234) centre (10.4529, -3.6142) ccw projected
  arc A358 (10.7054, -0.6234) -> (10.6662, -0.411) centre (6.6305, -1.2645) ccw projected
  arc A359 (10.6662, -0.411) -> (11.2682, -0.0269) centre (9.3642, 2.2934) ccw projected
  arc A360 (11.2682, -0.0269) -> (11.1971, 0.2141) centre (6.6305, -1.2645) ccw projected
  arc A361 (11.1971, 0.2141) -> (10.483, 0.2098) centre (10.8579, -2.7682) ccw projected
  arc A362 (10.483, 0.2098) -> (10.4006, 0.4094) centre (6.6305, -1.2645) ccw projected
  circle A363 centre (6.6305, -1.2645) radius 1.5
  circle A364 centre (-4.4104, -5.1099) radius 1.5
  circle A365 centre (-2.2201, 6.3744) radius 1.5
  constraints: 3 centre point, 3 coincident, 3 concentric
extrude "Extrusion2" add sketch "Skizze2" along normal blind 2 contours A0 | A121 | A242
